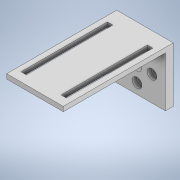
# Autodesk Inventor part: ServoESP32Base2
Saved by Autodesk Inventor 2020 (Build 240168000, 168)
## iProperties
Created: 2022-11-30
Part Number: ServoESP32Base2
Material: Generic
Document SubType Name: Modeling
Designer: agraa4529
Density: 1 g/cm^3
Appearance: Default
Author: agraa4529
## iProperties of the stored document _3DPrint.ipt
Created: 2022-12-02
Part Number: _3DPrint
Material: Generic
Document SubType Name: Modeling
Designer: agraa4529
Density: 1 g/cm^3
Appearance: Default
Author: agraa4529
Autodesk Inventor part; units mm, degrees
ref_plane "YZ Plane" through (0, 0, 0) normal (1, 0, 0) x (0, 1, 0)
ref_plane "XZ Plane" through (0, 0, 0) normal (0, 1, 0) x (-1, 0, 0)
ref_plane "XY Plane" through (0, 0, 0) normal (0, 0, 1) x (1, 0, 0)
sketch "Sketch1" plane through (0, 0, 0) normal (0, 0, 1) x (1, 0, 0)
  line L0 (-16, -16) -> (16, -16)
  line L1 (16, -16) -> (16, 16)
  line L2 (16, 16) -> (-16, 16)
  line L3 (-16, 16) -> (-16, -16)
  line L4 (-16, -16) -> (16, 16) construction
  line L5 (16, -16) -> (-16, 16) construction
  point P0 (0, 0)
  dimension "d1" = 32
  dimension "d2" = 32
  constraints: 12 end point, 2 midpoint, 2 parallel, 1 horizontal, 1 perpendicular
  measures "d1" distance of L2.end L1.end
  measures "d2" distance of L0.end L1.end
extrude "Extrusion1" add sketch "Sketch1" along normal blind 5
sketch "Sketch2" plane through (0, 0, 5) normal (0, 0, 1) x (1, 0, 0)
  line L0 (0, 0) -> (9.5, 0) construction
  circle A0 centre (9.5, 0) radius 1.5
  line L1 (0, 0) -> (0, 9.5) construction
  circle A1 centre (0, 9.5) radius 1.5
  line L2 (0, 0) -> (-9.5, 0) construction
  circle A2 centre (-9.5, 0) radius 1.5
  line L3 (0, 0) -> (0, -9.5) construction
  circle A3 centre (0, -9.5) radius 1.5
  dimension "d5" = 3
  dimension "d6" = 9.5
  dimension "d9" = 360
  constraints: 8 end point, 6 coincident, 4 centre point, 1 horizontal, 19 other
  measures "d5" diameter of A0
  measures "d6" distance of L0.start L0.end
extrude "Extrusion2" cut sketch "Sketch2" against normal blind 5
sketch "Sketch3" plane through (0, 0, 5) normal (0, 0, 1) x (1, 0, 0)
  circle A0 centre (0, 9.5) radius 1.5 projected
  circle A1 centre (0, 9.5) radius 3.1
  circle A2 centre (-9.5, 0) radius 3.1
  circle A3 centre (0, -9.5) radius 3.1
  circle A4 centre (9.5, 0) radius 3.1
  point P0 (0, 0)
  dimension "d13" = 6.2
  dimension "d16" = 360
  constraints: 4 centre point, 1 coincident, 9 other
  measures "d13" diameter of A1
extrude "Extrusion3" cut sketch "Sketch3" against normal blind 2.5
sketch "Sketch5" plane through (0, 0, 5) normal (0, 0, 1) x (1, 0, 0)
  circle A0 centre (0, 0) radius 3
  dimension "d25" = 6
  constraints: 1 centre point, 1 coincident
  measures "d25" diameter of A0
extrude "Extrusion5" cut sketch "Sketch5" against normal blind 10
sketch "Sketch8" plane through (0, 0, 0) normal (0, 0, -1) x (-1, 0, 0)
  line L0 (16, -16) -> (-16, -16) projected
  line L1 (-16, -16) -> (16, -16)
  line L2 (-16, 16) -> (16, 16) projected
  line L3 (-16, 16) -> (16, 16)
  line L4 (16, 16) -> (16, 19)
  line L5 (16, 19) -> (-16, 19)
  line L6 (-16, 19) -> (-16, 16)
  point P0 (0, 0)
  dimension "d32" = 32
  dimension "d33" = 3
  constraints: 10 end point, 2 horizontal, 2 parallel, 1 perpendicular
  measures "d32" distance of L4.end L5.end
  measures "d33" distance of L3.end L4.end
extrude "Extrusion6" add sketch "Sketch8" against normal blind 70
sketch "Sketch10" plane through (-16, 19, 0) normal (0, 1, 0) x (1, 0, 0)
  line L0 (16, 0) -> (16, -70) construction
  line L1 (32, -70) -> (0, -70) projected
  line L2 (27, -9.4577) -> (5, -9.4577) construction
  line L3 (5, -9.4577) -> (5, -60.5423) construction
  line L4 (5, -60.5423) -> (27, -60.5423) construction
  line L5 (27, -60.5423) -> (27, -9.4577) construction
  line L6 (27, -9.4577) -> (5, -60.5423) construction
  line L7 (5, -9.4577) -> (27, -60.5423) construction
  line L8 (27, -9.4577) -> (30.5, -9.4577)
  line L9 (30.5, -9.4577) -> (30.5, -64.4577)
  line L10 (30.5, -64.4577) -> (27, -64.4577)
  line L11 (27, -64.4577) -> (27, -9.4577)
  line L12 (5, -9.4577) -> (1.5, -9.4577)
  line L13 (1.5, -9.4577) -> (1.5, -64.4577)
  line L14 (1.5, -64.4577) -> (5, -64.4577)
  line L15 (5, -64.4577) -> (5, -9.4577)
  point P0 (16, -35)
  dimension "d41" = 22
  dimension "d42" = 3.5
  dimension "d43" = 3.5
  dimension "d44" = 55
  dimension "d45" = 55
  constraints: 30 end point, 6 parallel, 4 midpoint, 3 horizontal, 3 perpendicular
  measures "d41" distance of L4.end L3.end
  measures "d42" distance of L9.end L10.end
  measures "d43" distance of L14.end L13.end
  measures "d44" distance of L8.end L9.end
  measures "d45" distance of L12.end L13.end
extrude "Extrusion8" cut sketch "Sketch10" against normal blind 10
sketch "Sketch11" plane through (16, -16, 5) normal (1, 0, 0) x (0, 0, -1)
  line L0 (0, 0) -> (0, 32) projected
  line L1 (0, 32) -> (0, 0)
  line L2 (5, 0) -> (0, 0) projected
  line L3 (0, 0) -> (5, 0)
  line L4 (5, 0) -> (5, 35) projected
  line L5 (5, 0) -> (5, 35)
  line L6 (5, 35) -> (-65, 35) projected
  line L7 (5, 35) -> (-65, 35)
  line L8 (-65, 35) -> (-65, 32)
  line L9 (-65, 32) -> (0, 32)
  point P0 (5, 16)
  constraints: 12 end point, 5 perpendicular, 1 vertical
extrude "Extrusion9" add sketch "Sketch11" along normal blind 2
sketch "Sketch12" plane through (-16, -16, 0) normal (-1, 0, 0) x (0, 0, 1)
  line L0 (70, 32) -> (5, 32) projected
  line L1 (0, 0) -> (5, 0) projected
  line L2 (5, 32) -> (5, 0)
  line L3 (5, 0) -> (0, 0)
  line L4 (0, 35) -> (70, 35) projected
  line L5 (0, 0) -> (0, 35)
  line L6 (0, 35) -> (70, 35)
  line L7 (70, 35) -> (70, 32) projected
  line L8 (70, 35) -> (70, 32)
  line L9 (70, 32) -> (5, 32)
  point P0 (0, 16)
  constraints: 12 end point, 4 perpendicular, 2 collinear
extrude "Extrusion10" add sketch "Sketch12" along normal blind 2
body "Solid1"
